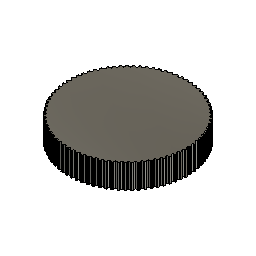
gear_79z (Autodesk Fusion 360 design; units mm, degrees)
Autodesk Fusion 360 part; units mm, degrees
sketch "Sketch1" plane through (0, 0, 0) normal (0, 0, 1) x (1, 0, 0) in component "gt2 pulley"
  circle A0 centre (0, 0) radius 25.1465 construction
  circle A1 centre (0, 0) radius 24.1425 construction
  line L0 (0, 0) -> (0, 25.1465) construction
  line L1 (0, 0) -> (0.9997, 25.1266) construction
  line L2 (0, 0) -> (1.4049, 25.1072) construction
  circle A2 centre (0, 0) radius 24.8925 construction
  arc A3 (0.3955, 24.7559) -> (0.4719, 24.4589) centre (1.3908, 24.8536) ccw
  circle A4 centre (0, 0) radius 24.7425 construction
  arc A5 (0.2477, 24.8912) -> (0, 24.8925) centre (0, 0) ccw
  arc A6 (0.3955, 24.7559) -> (0.2477, 24.8912) centre (0.2463, 24.7413) ccw
  arc A7 (0.4719, 24.4589) -> (0.9598, 24.1234) centre (0.9819, 24.678) ccw
  arc A8 (0, 24.8925) -> (-0.2477, 24.8912) centre (0, 0) ccw
  arc A9 (-0.2477, 24.8912) -> (-0.3955, 24.7559) centre (-0.2463, 24.7413) ccw
  arc A10 (-0.4719, 24.4589) -> (-0.3955, 24.7559) centre (-1.3908, 24.8536) ccw
  arc A11 (-0.9598, 24.1234) -> (-0.4719, 24.4589) centre (-0.9819, 24.678) ccw
  arc A12 (0.9598, 24.1234) -> (-0.9598, 24.1234) centre (0, 0) ccw
  point P0 (1.3908, 24.8536)
  point P1 (0, 24.8925)
  dimension "d18" = 50.293
  dimension "d19" = 2.278
  dimension "d22" = 1.004
  dimension "d24" = 0.75
  dimension "d26" = 1
  dimension "d27" = 0.15
  dimension "d28" = 0.15
  dimension "d47" = 0.555
  dimension "d52" = 3.812
  constraint coincident A0.centre A1.centre
  constraint coincident A0 L0.end
  constraint vertical L0
  constraint coincident A0 L1.end
  constraint coincident A0 L2.end
  constraint concentric A1 A2
  constraint coincident A1 A7.end
  constraint coincident L1 A7.end
  constraint coincident A2 P0
  constraint coincident L2 P0
  constraint coincident P0 A3.centre
  constraint coincident A2 P1
  constraint coincident L0 P1
  constraint concentric A2 A4
  constraint coincident P1 A5.end
  constraint coincident A4 A6.centre
  constraint coincident A3.start A6.start
  constraint tangent A3 A6
  constraint tangent A3 A7
  constraint symmetric L0 A7.end A11.start
  constraint symmetric L0 A3.start A9.end
  constraint symmetric L0 A3.end A10.start
  constraint symmetric L0 A3 A10
  constraint symmetric L0 A5.start A8.end
  constraint symmetric L0 P1 A5.end
  constraint symmetric L0 A5 A8
  constraint symmetric L0 A6 A9
  constraint symmetric L0 A7 A11
  constraint coincident A1 A11.start
  constraint tangent A1 A7
  constraint coincident L1 A7.centre
  measures "d18" diameter of A0
  measures "d19" angle of L0 L1
  measures "d22" distance of A0 A1
  measures "d24" distance of A1 A2
  measures "d26" radius of A3
  measures "d27" distance of A2 A4
  measures "d28" radius of A6
  measures "d47" radius of A7
extrude "Extrude1" add sketch "Sketch1" along normal blind 10 makes body 1
pattern_circular "C-Pattern1" count 79 over 360 about axis through (0, 0, 1.75) along (0, 0, 1) of bodies 1 makes body 2 at (-2.6615, 23.9953, 6.6667) makes body 3 at (-3.0851, 23.9445, 3.3333) makes body 4 at (-6.4287, 23.2708, 6.6667) makes body 5 at (-8.2572, 22.6865, 6.6667) makes body 6 at (-9.2512, 22.2996, 6.6667) makes body 7 at (-11.7465, 21.0922, 6.6667) makes body 8 at (-13.3851, 20.0922, 6.6667) makes body 9 at (-14.9391, 18.9653, 6.6667) makes body 10 at (-15.272, 18.6983, 6.6667) makes body 11 at (-17.3147, 16.8244, 6.6667) makes body 12 at (-18.9982, 14.8972, 6.6667) makes body 13 at (-20.1218, 13.3407, 6.6667) makes body 14 at (-20.3544, 12.983, 3.3333) makes body 15 at (-21.9809, 9.985, 6.6667) makes body 16 at (-22.7047, 8.2071, 6.6667) makes body 17 at (-23.2277, 6.5828, 6.6667) makes body 18 at (-23.394, 5.9647, 6.6667) makes body 19 at (-23.894, 3.455, 6.6667) makes body 20 at (-24.1057, 1.3328, 6.6667) makes body 21 at (-24.141, 0.2667, 3.3333) makes body 22 at (-24.0859, -1.6522, 3.3333) makes body 23 at (-23.8785, -3.5606, 6.6667) makes body 24 at (-23.5201, -5.4465, 3.3333) makes body 25 at (-22.7407, -8.1067, 6.6667) makes body 26 at (-22.3605, -9.1032, 3.3333) makes body 27 at (-21.5665, -10.851, 3.3333) makes body 28 at (-19.8221, -13.7819, 6.6667) makes body 29 at (-19.5755, -14.1301, 3.3333) makes body 30 at (-17.8267, -16.2809, 6.6667) makes body 31 at (-16.4768, -17.6458, 6.6667) makes body 32 at (-15.6813, -18.3564, 3.3333) makes body 33 at (-14.1733, -19.5442, 3.3333) makes body 34 at (-12.5757, -20.6085, 3.3333) makes body 35 at (-10.1305, -21.9142, 6.6667) makes body 36 at (-7.754, -22.8634, 6.6667) makes body 37 at (-5.913, -23.4072, 6.6667) makes body 38 at (-4.0346, -23.803, 6.6667) makes body 39 at (-3.6133, -23.8706, 3.3333) makes body 40 at (-0.2133, -24.1415, 6.6667) makes body 41 at (1.7054, -24.0822, 6.6667) makes body 42 at (2.1307, -24.0483, 3.3333) makes body 43 at (5.4984, -23.508, 6.6667) makes body 44 at (5.913, -23.4072, 6.6667) makes body 45 at (8.5572, -22.5751, 6.6667) makes body 46 at (9.546, -22.1751, 3.3333) makes body 47 at (11.2777, -21.3465, 3.3333) makes body 48 at (12.938, -20.383, 3.3333) makes body 49 at (15.1892, -18.7656, 6.6667) makes body 50 at (16.0033, -18.0763, 3.3333) makes body 51 at (17.9699, -16.1227, 6.6667) makes body 52 at (18.6645, -15.3133, 3.3333) makes body 53 at (19.8221, -13.7819, 3.3333) makes body 54 at (20.8545, -12.1635, 3.3333) makes body 55 at (22.3605, -9.1032, 6.6667) makes body 56 at (22.8115, -7.9054, 6.6667) makes body 57 at (23.1384, -6.8901, 3.3333) makes body 58 at (23.6127, -5.0299, 6.6667) makes body 59 at (24.0336, -2.2901, 6.6667) makes body 60 at (24.1113, -1.2262, 3.3333) makes body 61 at (24.1325, 0.6933, 3.3333) makes body 62 at (23.9236, 3.2437, 6.6667) makes body 63 at (23.718, 4.5071, 6.6667) makes body 64 at (23.285, 6.3772, 3.3333) makes body 65 at (22.4005, 9.0044, 6.6667) makes body 66 at (21.3216, 11.3248, 6.6667) makes body 67 at (20.3544, 12.983, 6.6667) makes body 68 at (19.7611, 13.8694, 6.6667) makes body 69 at (18.0409, 16.0432, 6.6667) makes body 70 at (16.7093, 17.4258, 6.6667) makes body 71 at (15.272, 18.6983, 6.6667) makes body 72 at (14.9391, 18.9653, 3.3333) makes body 73 at (12.1174, 20.8813, 6.6667) makes body 74 at (10.4201, 21.778, 6.6667) makes body 75 at (9.4479, 22.217, 6.6667) makes body 76 at (8.2572, 22.6865, 3.3333) makes body 77 at (4.9778, 23.6237, 6.6667) makes body 78 at (3.0851, 23.9446, 6.6667) makes body 79 at (2.6615, 23.9953, 3.3333)
sketch "Sketch2" plane through (0, 0, 10) normal (0, 0, 1) x (-1, 0, 0)
  arc A0 (-15.0281, -19.6766) -> (-14.9896, -19.8733) centre (-14.8993, -19.7535) ccw
  arc A1 (-14.9896, -19.8733) -> (-14.5912, -20.1676) centre (0, 0) ccw
  arc A2 (-14.5912, -20.1676) -> (-14.3918, -20.1466) centre (-14.5032, -20.0461) ccw
  arc A3 (-14.1539, -19.9531) -> (-14.3918, -20.1466) centre (-13.6494, -20.8165) ccw
  arc A4 (-13.5621, -19.9732) -> (-14.1539, -19.9531) centre (-13.8739, -20.4323) ccw
  arc A5 (-15.1061, -18.8325) -> (-13.5621, -19.9732) centre (0, 0) ccw
  arc A6 (-14.9131, -19.3923) -> (-15.1061, -18.8325) centre (-15.4534, -19.2655) ccw
  arc A7 (-15.0281, -19.6766) -> (-14.9131, -19.3923) centre (-15.8866, -19.1638) ccw
  circle A8 centre (0, 0) radius 24.1425
  constraint concentric A1 A8
extrude "Extrude2" add sketch "Sketch2" against normal blind 10 contours A5 A8 bodies 1 2 3 4 5 6 7 8 9 10 11 12 13 14 15 16 17 18 19 20 21 22 23 24 25 26 27 28 29 30 31 32 33 34 35 36 37 38 39 40 41 42 43 44 45 46 47 48 49 50 51 52 53 54 55 56 57 58 59 60 61 62 63 64 65 66 67 68 69 70 71 72 73 74 75 76 77 78 79
extrude "Extrude4" [suppressed] in component "gt2 pulley"
pattern_circular "C-Pattern7" [suppressed] in component "gt2 pulley"
extrude "Extrude3" [suppressed] in component "gt2 pulley"
pattern_circular "C-Pattern6" [suppressed] in component "gt2 pulley"
extrude "Extrude2'" [suppressed] in component "gt2 pulley"
pattern_circular "C-Pattern5" [suppressed] in component "gt2 pulley"
extrude "Extrude1'" [suppressed] in component "gt2 pulley"
pattern_circular "C-Pattern4" [suppressed] in component "gt2 pulley"
pattern_circular "C-Pattern3" [suppressed] in component "gt2 pulley"
pattern_circular "C-Pattern2" [suppressed] in component "gt2 pulley"
pattern_circular "C-Pattern1'" [suppressed] in component "gt2 pulley"
copy_body "Body->Comp1" [suppressed] in component "Component"
copy_body "Body->Comp2" [suppressed] in component "Component'"
copy_body "Body->Comp3" [suppressed] in component "Component''"
copy_body "Body->Comp4" [suppressed] in component "Component'''"
copy_body "Body->Comp5" [suppressed] in component "Component''''"
copy_body "Body->Comp6" [suppressed] in component "Component'''''"
copy_body "Body->Comp7" [suppressed] in component "Component''''''"
copy_body "Body->Comp8" [suppressed] in component "Component'''''''"
copy_body "Body->Comp9" [suppressed] in component "Component''''''''"
copy_body "Body->Comp10" [suppressed] in component "Component'''''''''"
copy_body "Body->Comp11" [suppressed] in component "Component''''''''''"
copy_body "Body->Comp12" [suppressed] in component "Component'''''''''''"
copy_body "Body->Comp13" [suppressed] in component "Component''''''''''''"
copy_body "Body->Comp14" [suppressed] in component "Component'''''''''''''"
copy_body "Body->Comp15" [suppressed] in component "Component''''''''''''''"
copy_body "Body->Comp16" [suppressed] in component "Component'''''''''''''''"
copy_body "Body->Comp17" [suppressed] in component "Component''''''''''''''''"
copy_body "Body->Comp18" [suppressed] in component "Component'''''''''''''''''"
copy_body "Body->Comp19" [suppressed] in component "Component''''''''''''''''''"
copy_body "Body->Comp20" [suppressed] in component "Component'''''''''''''''''''"
component "gt2 pulley" placed x (1, 0, 0) y (0, 1, 0) z (0, 0, 1) at (0, 0, 0)
equation "NumTeeth = 79" comment "min 20"
equation "ToothPitch = 2 mm"
equation "PullyDia = NumTeeth * ToothPitch / PI"
equation "ToothAng = ( ( 360 / NumTeeth ) * 1 deg )"
equation "TransOffsetAngle = ToothAng * 0.2"
equation "Sholulder_Radius = 0.15 mm"
equation "Root_Radius = 0.555 mm"
equation "TransRadius = 1 mm"
equation "ToolHeight = 0.75 mm"
equation "PLD = 0.254 mm"
equation "d18 = PullyDia"
equation "d19 = ToothAng / 2"
equation "d22 = PLD + ToolHeight"
equation "d24 = ToolHeight"
equation "d26 = TransRadius"
equation "d27 = Sholulder_Radius"
equation "d31 = NumTeeth"
equation "d33 = NumTeeth"
equation "d35 = NumTeeth"
equation "d37 = NumTeeth"
equation "d41 = NumTeeth"
equation "d45 = NumTeeth"
equation "d47 = Root_Radius"
equation "d50 = NumTeeth"
